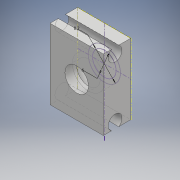
# Autodesk Inventor part: slider-top-anker
Saved by Autodesk Inventor 2018 (Build 220112000, 112)
## iProperties
Created: 2025-09-13
Part Number: slider-top-anker
Material: Generic
Document SubType Name: Modeling
Designer: neo
Density: 1 g/cm^3
Appearance: Default
Author: neo
Autodesk Inventor part; units mm, degrees
ref_plane "YZ Plane" through (0, 0, 0) normal (1, 0, 0) x (0, 1, 0)
ref_plane "XZ Plane" through (0, 0, 0) normal (0, 1, 0) x (-1, 0, 0)
ref_plane "XY Plane" through (0, 0, 0) normal (0, 0, 1) x (1, 0, 0)
sketch "Sketch1" plane through (0, 0, 0) normal (0, 0, 1) x (1, 0, 0)
  line L0 (-7.6738, 6.4198) -> (5.9262, 6.4198)
  line L1 (5.9262, 6.4198) -> (5.9262, -0.5802)
  line L2 (5.9262, -0.5802) -> (-7.6738, -0.5802)
  line L3 (-7.6738, -0.5802) -> (-7.6738, 6.4198)
  point P0 (0, 0)
  dimension "d0" = 7
  dimension "d1" = 13.6
  constraints: 8 end point, 2 parallel, 1 horizontal, 1 perpendicular
  measures "d0" distance of L2.end L0.start
  measures "d1" distance of L0.start L0.end
extrude "Extrusion1" add sketch "Sketch1" along normal blind 18
sketch "Sketch2" plane through (5.9262, -0.5802, 0) normal (1, 0, 0) x (0, 0, -1)
  line L0 (-9, 7.1029) -> (-9, -3.9254)
  line L1 (-18.4841, 3) -> (1.1812, 3) construction
  circle A0 centre (-16.5, 3) radius 1.75
  circle A1 centre (-1.5, 3) radius 1.75
  line L2 (0, 7) -> (0, 0) construction
  line L3 (0, 7) -> (-18, 7) construction
  line L4 (-18, 0) -> (-18, 7) construction
  line L5 (0, 0) -> (-18, 0) construction
  line L6 (0, 7) -> (-18, 7) construction
  line L7 (-9, 7) -> (-9, 9.8874) construction
  point P0 (0, 0.5802)
  dimension "d4" = 3.5
  dimension "d6" = 15
  dimension "d23" = 3
  constraints: 6 end point, 2 centre point, 2 point on line, 2 vertical, 1 collinear, 1 horizontal, 1 midpoint, 1 other
  measures "d4" diameter of A0
  measures "d6" diameter of A0.centre L0
  measures "d23" distance between parallel lines of L5 L1
extrude "Extrusion2" cut sketch "Sketch2" against normal through all
sketch "Sketch3" plane through (-7.6738, 6.4198, 0) normal (0, 1, 0) x (1, 0, 0)
  line L0 (13.6, -18) -> (0, -18) projected
  line L1 (6.8, -18) -> (6.8, 8.3018)
  line L2 (0, 0) -> (0, -18) projected
  line L3 (0, -9) -> (13.6, -9)
  line L4 (13.6, 0) -> (13.6, -18) projected
  circle A0 centre (6.8, -9) radius 3
  circle A1 centre (6.8, -9) radius 4.1
  point P0 (7.6738, 0)
  dimension "d9" = 6
  dimension "d10" = 8.2
  constraints: 4 end point, 4 midpoint, 2 centre point, 1 coincident, 1 vertical
  measures "d9" diameter of A0
  measures "d10" diameter of A1
extrude "bearing depth 2mm" cut sketch "Sketch3" against normal blind 4 contours A1 L3 A0 L1 | L1 A0 L3 A1 | L3 A0 L1 A1 | A1 L1 A0 L3
extrude "Extrusion4" cut sketch "Sketch3" against normal up to surface (7 mm away) contours A0 L3 L1 | L1 L3 A0 | L3 L1 A0 | L3 A0 L1
body "Solid1"
